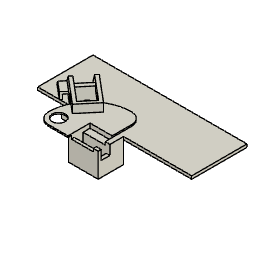
sorting_mechanism_platform (Autodesk Fusion 360 design; units mm, degrees)
Autodesk Fusion 360 part; units mm, degrees
note: some values were not read from the file. Set by a fixed rule: which sketch regions a step uses.
sketch "Sketch1" plane through (0, 0, 0) normal (0, 0, 1) x (1, 0, 0)
  line L0 (0, 0) -> (212, 0)
  line L1 (212, 0) -> (212, 78)
  line L2 (212, 78) -> (0, 78)
  line L3 (0, 78) -> (0, 0)
  dimension "d1" = 212
  dimension "d2" = 78
  constraint horizontal L0
  constraint vertical L1
  constraint horizontal L2
  constraint vertical L3
  constraint coincident L0.start L3.end
  measures "d1" distance of L0.start L0.end
  measures "d2" distance of L0.end L1.end
extrude "Extrude1" add sketch "Sketch1" along normal blind 4 makes body 1
sketch "Sketch2" plane through (0, 0, 4) normal (0, 0, 1) x (-1, 0, 0)
  line L0 (0, -78) -> (0, 0)
  line L1 (0, 0) -> (-212, 0)
  line L2 (-212, 0) -> (-212, -78)
  line L3 (-212, -78) -> (0, -78)
  line L4 (-31.7137, -41.9046) -> (-37.7137, -41.9046)
  line L5 (-37.7137, -41.9046) -> (-37.7137, -11.9046)
  line L6 (-37.7137, -11.9046) -> (-31.7137, -11.9046)
  line L7 (-31.7137, -11.9046) -> (-31.7137, -41.9046)
  dimension "d7" = 30
  dimension "d32" = 6
  constraint horizontal L4
  constraint vertical L5
  constraint horizontal L6
  constraint vertical L7
  measures "d7" distance of L4.start L6.end
  measures "d32" distance of L4.start L4.end
extrude "Extrude2" add sketch "Sketch2" along normal blind 12 contours L4 L5 L6 L7 bodies 1
sketch "Sketch4" plane through (0, 0, 16) normal (0, 0, 1) x (-1, 0, 0)
  line L0 (-31.7137, -11.9046) -> (-37.7137, -11.9046)
  line L1 (-37.7137, -11.9046) -> (-37.7137, -41.9046)
  line L2 (-37.7137, -41.9046) -> (-31.7137, -41.9046)
  line L3 (-31.7137, -41.9046) -> (-31.7137, -11.9046)
  line L4 (-31.7137, -41.9046) -> (-71.7137, -41.9046)
  line L5 (-71.7137, -41.9046) -> (-71.7137, -11.9046)
  line L6 (-71.7137, -11.9046) -> (-31.7137, -11.9046)
  line L7 (-31.7137, -11.9046) -> (-31.7137, -41.9046)
  dimension "d33" = 40
  constraint horizontal L4
  constraint vertical L5
  constraint horizontal L6
  constraint vertical L7
  constraint coincident L2.end L3.start
  constraint collinear L0 L6
  measures "d33" distance of L5 L7
extrude "Extrude3" add sketch "Sketch4" along normal blind 11 bodies 1
sketch "Sketch5" plane through (0, 0, 27) normal (0, 0, 1) x (-1, 0, 0)
  line L0 (-31.7137, -11.9046) -> (-71.7137, -11.9046)
  line L1 (-71.7137, -11.9046) -> (-71.7137, -41.9046)
  line L2 (-71.7137, -41.9046) -> (-31.7137, -41.9046)
  line L3 (-31.7137, -41.9046) -> (-31.7137, -11.9046)
  line L4 (-67.4138, -16.4046) -> (-37.7137, -16.4046)
  line L5 (-37.7137, -16.4046) -> (-37.7137, -37.4046)
  line L6 (-37.7137, -37.4046) -> (-67.4138, -37.4046)
  line L7 (-67.4138, -37.4046) -> (-67.4138, -16.4046)
  dimension "d14" = 21
  dimension "d15" = 4.5
  dimension "d34" = 6
  constraint horizontal L4
  constraint vertical L5
  constraint horizontal L6
  constraint vertical L7
  measures "d14" distance of L4.start L6.end
  measures "d15" distance of L2 L6
  measures "d34" distance of L3 L5
extrude "Extrude4" cut sketch "Sketch5" against normal blind 11 contours L4 L5 L6 L7 bodies 1
sketch "Sketch7" plane through (0, 0, 27) normal (0, 0, 1) x (-1, 0, 0)
  line L0 (-37.7137, -16.4046) -> (-37.7137, -37.4046)
  line L1 (-37.7137, -37.4046) -> (-67.4138, -37.4046)
  line L2 (-67.4138, -16.4046) -> (-37.7137, -16.4046)
  line L3 (-31.7137, -11.9046) -> (-71.7137, -11.9046)
  line L4 (-71.7137, -11.9046) -> (-71.7137, -41.9046)
  line L5 (-71.7137, -41.9046) -> (-31.7137, -41.9046)
  line L6 (-31.7137, -41.9046) -> (-31.7137, -11.9046)
  line L7 (-37.7137, -16.4046) -> (-31.7137, -16.4046)
  line L8 (-31.7137, -16.4046) -> (-31.7137, -37.4046)
  line L9 (-31.7137, -37.4046) -> (-37.7137, -37.4046)
  line L10 (-37.7137, -37.4046) -> (-37.7137, -16.4046)
  line L11 (-67.4138, -37.4046) -> (-67.4138, -16.4046)
  constraint horizontal L7
  constraint vertical L8
  constraint horizontal L9
  constraint vertical L10
  constraint coincident L6 L8.end
  constraint coincident L0.start L2.end
  constraint collinear L1 L9
extrude "Extrude5" cut sketch "Sketch7" against normal blind 4 contours L0 L6 L7 L8 L9 L10 bodies 1
sketch "Sketch8" plane through (0, 11.9046, 0) normal (0, -1, 0) x (1, 0, 0)
  line L0 (31.7137, 4) -> (37.7137, 4)
  line L1 (37.7137, 4) -> (37.7137, 16)
  line L2 (37.7137, 16) -> (71.7137, 16)
  line L3 (71.7137, 16) -> (71.7137, 27)
  line L4 (71.7137, 27) -> (31.7137, 27)
  line L5 (31.7137, 27) -> (31.7137, 4)
  line L6 (31.7137, 27) -> (24.7137, 27)
  line L7 (31.7137, 27) -> (31.7137, 4)
  line L8 (31.7137, 4) -> (4.7137, 4)
  line L9 (24.7137, 27) -> (4.7137, 4)
  dimension "d42" = 7
  dimension "d43" = 27
  constraint coincident L4.end L5.start
  constraint perpendicular L5 L6
  constraint coincident L0.start L5.end
  constraint perpendicular L7 L8
  measures "d42" distance of L4.end L6.end
  measures "d43" distance of L0.start L8.end
extrude "Extrude6" add sketch "Sketch8" against normal blind 4.5 contours L5 L6 L7 L8 L9 bodies 1
sketch "Sketch9" plane through (0, 41.9046, 0) normal (0, 1, 0) x (-1, 0, 0)
  line L0 (-37.7137, 4) -> (-31.7137, 4)
  line L1 (-31.7137, 4) -> (-31.7137, 27)
  line L2 (-31.7137, 27) -> (-71.7137, 27)
  line L3 (-71.7137, 27) -> (-71.7137, 16)
  line L4 (-71.7137, 16) -> (-37.7137, 16)
  line L5 (-37.7137, 16) -> (-37.7137, 4)
  line L6 (-31.7137, 27) -> (-24.7137, 27)
  line L7 (-31.7137, 27) -> (-31.7137, 4)
  line L8 (-31.7137, 4) -> (-4.7137, 4)
  line L9 (-24.7137, 27) -> (-4.7137, 4)
  dimension "d44" = 7
  dimension "d45" = 27
  constraint coincident L1.end L2.start
  constraint perpendicular L1 L6
  constraint coincident L0.end L1.start
  constraint perpendicular L1 L8
  measures "d44" distance of L1.end L6.end
  measures "d45" distance of L0.end L8.end
extrude "Extrude7" add sketch "Sketch9" against normal blind 4.5 contours L1 L6 L7 L8 L9 bodies 1
sketch "Sketch10" plane through (67.4138, 0, 0) normal (-1, 0, 0) x (0, -1, 0)
  line L0 (-16.4046, 27) -> (-37.4046, 27)
  line L1 (-37.4046, 27) -> (-37.4046, 16)
  line L2 (-16.4046, 16) -> (-16.4046, 27)
  line L3 (-29.9046, 25) -> (-23.9046, 25)
  line L4 (-23.9046, 25) -> (-23.9046, 22)
  line L5 (-23.9046, 22) -> (-29.9046, 22)
  line L6 (-29.9046, 22) -> (-29.9046, 27)
  line L7 (-37.4046, 16) -> (-16.4046, 16)
  dimension "d24" = 3
  dimension "d25" = 6
  dimension "d28" = 7.5
  dimension "d29" = 7.5
  dimension "d30" = 2
  constraint vertical L4
  constraint horizontal L5
  constraint vertical L6
  constraint coincident L0 L6.end
  constraint coincident L6 L3.start
  constraint perpendicular L3 L6
  measures "d24" distance of L3.end L4.end
  measures "d25" distance of L4.end L5.end
  measures "d28" distance of L1 L6
  measures "d29" distance of L2 L4
  measures "d30" distance of L0 L3
extrude "Extrude8" add sketch "Sketch10" along normal blind 4 contours L3 L4 L5 L6 bodies 1
sketch "Sketch11" plane through (0, 0, 4) normal (0, 0, 1) x (-1, 0, 0)
  line L0 (-31.7137, -37.4046) -> (-4.7137, -37.4046)
  line L1 (-4.7137, -37.4046) -> (-4.7137, -41.9046)
  line L2 (-4.7137, -41.9046) -> (-37.7137, -41.9046)
  line L3 (-37.7137, -41.9046) -> (-37.7137, -11.9046)
  line L4 (-37.7137, -11.9046) -> (-4.7137, -11.9046)
  line L5 (-4.7137, -11.9046) -> (-4.7137, -16.4046)
  line L6 (-4.7137, -16.4046) -> (-31.7137, -16.4046)
  line L7 (-31.7137, -16.4046) -> (-31.7137, -37.4046)
  line L8 (0, -78) -> (0, 0)
  line L9 (0, 0) -> (-212, 0)
  line L10 (-212, 0) -> (-212, -78)
  line L11 (-212, -78) -> (0, -78)
  circle A0 centre (-98, -18.5) radius 10
  dimension "d46" = 20
  dimension "d47" = 59.5
  dimension "d50" = 114
  measures "d46" diameter of A0
  measures "d47" distance of L11 A0.centre
  measures "d50" distance of L10 A0.centre
extrude "Extrude9" add sketch "Sketch11" along normal blind 2 contours A0 bodies 1
sketch "Sketch12" plane through (0, 0, 0) normal (0, 0, -1) x (1, 0, 0)
  line L0 (0, 0) -> (0, -78)
  line L1 (0, -78) -> (212, -78)
  line L2 (212, -78) -> (212, 0)
  line L3 (212, 0) -> (0, 0)
  line L4 (77.5, 0) -> (118.5, 0)
  line L5 (118.5, 0) -> (118.5, -4)
  line L6 (118.5, -4) -> (77.5, -4)
  line L7 (77.5, -4) -> (77.5, 0)
  circle A0 centre (98, -18.5) radius 10
  dimension "d60" = 4
  dimension "d66" = 20.5
  dimension "d67" = 41
  constraint horizontal L4
  constraint vertical L5
  constraint horizontal L6
  constraint vertical L7
  constraint coincident L3 L4.start
  measures "d60" distance of L4.end L5.end
  measures "d66" distance of L5 A0.centre
  measures "d67" distance of L5.end L6.end
extrude "Extrude10" add sketch "Sketch12" along normal blind 29 contours L3 L4 L5 L6 L7 bodies 1
sketch "Sketch18" plane through (0, 0, 0) normal (0, -1, 0) x (1, 0, 0)
  line L0 (0, 0) -> (77.5, 0)
  line L1 (77.5, 0) -> (77.5, -29)
  line L2 (77.5, -29) -> (118.5, -29)
  line L3 (118.5, -29) -> (118.5, 0)
  line L4 (118.5, 0) -> (212, 0)
  line L5 (212, 0) -> (212, 4)
  line L6 (212, 4) -> (0, 4)
  line L7 (0, 4) -> (0, 0)
  line L8 (77.5, -29) -> (118.5, -29)
  line L9 (118.5, -29) -> (118.5, -25)
  line L10 (118.5, -25) -> (77.5, -25)
  line L11 (77.5, -25) -> (77.5, -29)
  dimension "d61" = 4
  constraint horizontal L8
  constraint vertical L9
  constraint horizontal L10
  constraint vertical L11
  constraint coincident L3 L9.end
  constraint coincident L1.end L2.start
  measures "d61" distance of L2.end L9.end
extrude "Extrude14" add sketch "Sketch18" along normal blind 30.5 contours L1 L2 L3 L8 L9 L10 L11 bodies 1
sketch "Sketch19" plane through (118.5, 0, 0) normal (1, 0, 0) x (0, 1, 0)
  line L0 (4, 0) -> (0, 0)
  line L1 (0, 0) -> (0, -25)
  line L2 (0, -25) -> (-30.5, -25)
  line L3 (-30.5, -25) -> (-30.5, -29)
  line L4 (-30.5, -29) -> (4, -29)
  line L5 (4, -29) -> (4, 0)
  line L6 (-30.5, -25) -> (0, -25)
  line L7 (0, -25) -> (0, 4)
  line L8 (0, 4) -> (-30.5, 4)
  line L9 (-30.5, 4) -> (-30.5, -25)
  line L10 (-30.5, -25) -> (0, -25)
  line L11 (0, -25) -> (0, 4)
  constraint coincident L2.end L3.start
  constraint coincident L1.end L2.start
  constraint perpendicular L0 L7
  constraint horizontal L8
  constraint vertical L9
  constraint horizontal L10
  constraint vertical L11
extrude "Extrude15" add sketch "Sketch19" against normal blind 41 contours L1 L2 L6 L7 L8 L9 L10 L11 bodies 1
sketch "Sketch21" plane through (0, 0, 4) normal (0, 0, 1) x (-1, 0, 0)
  circle A0 centre (-98, -18.5) radius 10
  line L0 (-31.7137, -37.4046) -> (-4.7137, -37.4046)
  line L1 (-4.7137, -37.4046) -> (-4.7137, -41.9046)
  line L2 (-4.7137, -41.9046) -> (-37.7137, -41.9046)
  line L3 (-37.7137, -41.9046) -> (-37.7137, -11.9046)
  line L4 (-37.7137, -11.9046) -> (-4.7137, -11.9046)
  line L5 (-4.7137, -11.9046) -> (-4.7137, -16.4046)
  line L6 (-4.7137, -16.4046) -> (-31.7137, -16.4046)
  line L7 (-31.7137, -16.4046) -> (-31.7137, -37.4046)
  line L8 (0, -78) -> (0, 0)
  line L9 (0, 0) -> (-77.5, 0)
  line L10 (-212, 0) -> (-212, -78)
  line L11 (-212, -78) -> (0, -78)
  circle A1 centre (-98, 24) radius 56.5
  line L12 (-98, 24) -> (-113, 24)
  line L13 (-113, 24) -> (-113, -32.5)
  line L14 (-113, -32.5) -> (-98, -32.5)
  line L15 (-98, -32.5) -> (-98, 24)
  line L16 (-98, 24) -> (-41.5, 24)
  line L17 (-41.5, 24) -> (-41.5, 39)
  line L18 (-41.5, 39) -> (-98, 39)
  line L19 (-98, 39) -> (-98, 24)
  line L20 (-113, 24) -> (-98, 24)
  line L21 (-98, 24) -> (-98, 39)
  line L22 (-98, 39) -> (-113, 39)
  line L23 (-113, 39) -> (-113, 24)
  line L24 (-77.5, 0) -> (-77.5, 30.5)
  line L25 (-77.5, 30.5) -> (-118.5, 30.5)
  line L26 (-118.5, 30.5) -> (-118.5, 0)
  line L27 (-118.5, 0) -> (-212, 0)
  dimension "d72" = 114
  dimension "d73" = 114
  dimension "d74" = 113
  dimension "d75" = 42.5
  dimension "d76" = 56.5
  dimension "d77" = 56.5
  dimension "d78" = 15
  dimension "d79" = 15
  constraint horizontal L12
  constraint vertical L13
  constraint horizontal L14
  constraint vertical L15
  constraint coincident A1.centre L12.start
  constraint horizontal L16
  constraint vertical L17
  constraint horizontal L18
  constraint vertical L19
  constraint horizontal L20
  constraint vertical L21
  constraint horizontal L22
  constraint vertical L23
  measures "d72" distance of A0.centre L10
  measures "d73" distance of L10 A1.centre
  measures "d74" diameter of A1
  measures "d75" distance of A0.centre A1.centre
  measures "d76" distance of L12.end L13.end
  measures "d77" distance of L17.end L18.end
  measures "d78" distance of L13.end L14.end
  measures "d79" distance of L16.end L17.end
extrude "Extrude17" add sketch "Sketch21" along normal blind 2 contours A0 L9 A1 L15 L16 L24 | A0 A1 L12 L13 L15 L20 | L16 L19 L21 L24 L25 | L12 L19 L20 L21 L23 L25 | A1 L13 L14 | A1 L16 L18 L19 L21 L24 L25 | L9 A1 L16 L24 | L19 L21 L22 L23 L25 | A1 L17 L18 bodies 1
fillet "Fillet1" radius 15 2 edges at (41.5, -39, 5) (113, 32.5, 5) on bodies 1
sketch "Sketch22" plane through (0, 0, 6) normal (0, 0, 1) x (-1, 0, 0)
  arc A0 (-113, -17.5) -> (-98, -32.5) centre (-98, -17.5) ccw
  arc A1 (-98, -32.5) -> (-41.5, 24) centre (-98, 24) ccw
  arc A2 (-41.5, 24) -> (-56.5, 39) centre (-56.5, 24) ccw
  line L0 (-56.5, 39) -> (-113, 39)
  line L1 (-113, 39) -> (-113, -17.5)
  line L2 (-113, 0) -> (-83, 0)
  line L3 (-83, 0) -> (-83, 39)
  line L4 (-83, 39) -> (-113, 39)
  line L5 (-113, 39) -> (-113, 0)
  line L6 (-77.5, -4) -> (-118.5, -4)
  line L7 (-118.5, -4) -> (-118.5, 30.5)
  line L8 (-118.5, 30.5) -> (-77.5, 30.5)
  line L9 (-77.5, 30.5) -> (-77.5, -4)
  line L10 (-113, -17.5) -> (-113, 30.5)
  line L11 (-118.5, 0) -> (-212, 0)
  line L12 (-212, 0) -> (-212, -78)
  line L13 (-212, -78) -> (0, -78)
  line L14 (0, -78) -> (0, 0)
  line L15 (0, 0) -> (-46.8507, 0)
  arc A3 (-98, -32.5) -> (-46.8507, 0) centre (-98, 24) ccw
  arc A4 (-113, -17.5) -> (-98, -32.5) centre (-98, -17.5) ccw
  line L16 (-31.7137, -37.4046) -> (-4.7137, -37.4046)
  line L17 (-4.7137, -37.4046) -> (-4.7137, -41.9046)
  line L18 (-4.7137, -41.9046) -> (-37.7137, -41.9046)
  line L19 (-37.7137, -41.9046) -> (-37.7137, -11.9046)
  line L20 (-37.7137, -11.9046) -> (-4.7137, -11.9046)
  line L21 (-4.7137, -11.9046) -> (-4.7137, -16.4046)
  line L22 (-4.7137, -16.4046) -> (-31.7137, -16.4046)
  line L23 (-31.7137, -16.4046) -> (-31.7137, -37.4046)
  line L24 (0, 0) -> (-46.8507, 0)
  line L25 (-118.5, 0) -> (-212, 0)
  line L26 (-113, 30.5) -> (-118.5, 30.5)
  line L27 (-118.5, 30.5) -> (-118.5, 0)
  line L28 (-83, 0) -> (-118.5, 0)
  line L29 (-118.5, 0) -> (-118.5, 9)
  line L30 (-118.5, 9) -> (-83, 9)
  line L31 (-83, 9) -> (-83, 0)
  dimension "d84" = 32.5
  dimension "d95" = 5.5
  dimension "d112" = 9
  constraint horizontal L2
  constraint horizontal L4
  constraint vertical L5
  constraint coincident L0 L3.end
  constraint coincident L1 L2.start
  constraint horizontal L28
  constraint vertical L29
  constraint horizontal L30
  constraint vertical L31
  constraint coincident L7 L29.end
  measures "d84" distance of A0.end L2
  measures "d95" distance of L3 L9
  measures "d112" distance of L2 L30
extrude "Extrude18" cut sketch "Sketch22" against normal blind 2 contours L1 L3 L5 L8 L10 L30 | L0 L1 L3 L4 L5 L8 bodies 1
sketch "Sketch23" plane through (0, 0, 6) normal (0, 0, 1) x (-1, 0, 0)
  line L0 (-83, 39) -> (-83, 9)
  line L1 (-113, 9) -> (-113, -17.5)
  arc A0 (-113, -17.5) -> (-98, -32.5) centre (-98, -17.5) ccw
  arc A1 (-98, -32.5) -> (-41.5, 24) centre (-98, 24) ccw
  arc A2 (-41.5, 24) -> (-56.5, 39) centre (-56.5, 24) ccw
  line L2 (-56.5, 39) -> (-83, 39)
  circle A3 centre (-55.5, 24) radius 9
  line L3 (-83, 9) -> (-113, 9)
  dimension "d89" = 18
  dimension "d90" = 15
  dimension "d91" = 14
  measures "d89" diameter of A3
  measures "d90" distance of L2 A3.centre
  measures "d91" distance of A1.end A3.centre
extrude "Extrude19" cut sketch "Sketch23" against normal blind 2 contours A3 bodies 1
sketch "Sketch24" plane through (0, 0, 4) normal (0, 0, 1) x (-1, 0, 0)
  line L0 (-113, -17.5) -> (-113, 9)
  line L1 (-83, 9) -> (-83, 30.5)
  line L2 (-83, 30.5) -> (-118.5, 30.5)
  line L3 (-118.5, 30.5) -> (-118.5, 0)
  line L4 (-118.5, 0) -> (-212, 0)
  line L5 (-212, 0) -> (-212, -78)
  line L6 (-212, -78) -> (0, -78)
  line L7 (0, -78) -> (0, 0)
  line L8 (0, 0) -> (-46.8507, 0)
  arc A0 (-98, -32.5) -> (-46.8507, 0) centre (-98, 24) ccw
  arc A1 (-113, -17.5) -> (-98, -32.5) centre (-98, -17.5) ccw
  line L9 (-31.7137, -37.4046) -> (-4.7137, -37.4046)
  line L10 (-4.7137, -37.4046) -> (-4.7137, -41.9046)
  line L11 (-4.7137, -41.9046) -> (-37.7137, -41.9046)
  line L12 (-37.7137, -41.9046) -> (-37.7137, -11.9046)
  line L13 (-37.7137, -11.9046) -> (-4.7137, -11.9046)
  line L14 (-4.7137, -11.9046) -> (-4.7137, -16.4046)
  line L15 (-4.7137, -16.4046) -> (-31.7137, -16.4046)
  line L16 (-31.7137, -16.4046) -> (-31.7137, -37.4046)
  line L17 (-83, 30.5) -> (-114.5, 30.5)
  line L18 (-114.5, 30.5) -> (-114.5, 18.5)
  line L19 (-114.5, 18.5) -> (-83, 18.5)
  line L20 (-83, 18.5) -> (-83, 30.5)
  line L21 (-113, 9) -> (-83, 9)
  dimension "d96" = 4
  dimension "d98" = 12
  constraint horizontal L17
  constraint vertical L18
  constraint horizontal L19
  constraint vertical L20
  constraint coincident L2 L1.end
  constraint collinear L1 L20
  measures "d96" distance of L3 L18
  measures "d98" distance of L17.end L18.end
extrude "Extrude20" cut sketch "Sketch24" against normal blind 29 contours L1 L2 L17 L18 L19 L20 bodies 1
sketch "Sketch25" plane through (0, -30.5, 0) normal (0, -1, 0) x (1, 0, 0)
  line L0 (83, -25) -> (83, 4)
  line L1 (83, 4) -> (77.5, 4)
  line L2 (77.5, 4) -> (77.5, -29)
  line L3 (77.5, -29) -> (118.5, -29)
  line L4 (118.5, -29) -> (118.5, 4)
  line L5 (118.5, 4) -> (114.5, 4)
  line L6 (114.5, 4) -> (114.5, -25)
  line L7 (114.5, -25) -> (83, -25)
  line L8 (77.5, -29) -> (118.5, -29)
  line L9 (118.5, -29) -> (118.5, 4)
  line L10 (118.5, 4) -> (77.5, 4)
  line L11 (77.5, 4) -> (77.5, -29)
  constraint horizontal L8
  constraint vertical L9
  constraint horizontal L10
  constraint vertical L11
  constraint coincident L4.end L5.start
  constraint coincident L2.end L3.start
extrude "Extrude21" add sketch "Sketch25" along normal blind 4 bodies 1
sketch "Sketch26" plane through (0, 0, 4) normal (0, 0, 1) x (-1, 0, 0)
  line L0 (-31.7137, -37.4046) -> (-4.7137, -37.4046)
  line L1 (-4.7137, -37.4046) -> (-4.7137, -41.9046)
  line L2 (-4.7137, -41.9046) -> (-37.7137, -41.9046)
  line L3 (-37.7137, -41.9046) -> (-37.7137, -11.9046)
  line L4 (-37.7137, -11.9046) -> (-4.7137, -11.9046)
  line L5 (-4.7137, -11.9046) -> (-4.7137, -16.4046)
  line L6 (-4.7137, -16.4046) -> (-31.7137, -16.4046)
  line L7 (-31.7137, -16.4046) -> (-31.7137, -37.4046)
  line L8 (-83, 18.5) -> (-114.5, 18.5)
  line L9 (-114.5, 18.5) -> (-114.5, 30.5)
  line L10 (-114.5, 30.5) -> (-83, 30.5)
  line L11 (-83, 30.5) -> (-83, 34.5)
  line L12 (-83, 34.5) -> (-118.5, 34.5)
  line L13 (-118.5, 34.5) -> (-118.5, 0)
  line L14 (-118.5, 0) -> (-212, 0)
  line L15 (-212, 0) -> (-212, -78)
  line L16 (-212, -78) -> (0, -78)
  line L17 (0, -78) -> (0, 0)
  line L18 (0, 0) -> (-46.8507, 0)
  arc A0 (-98, -32.5) -> (-46.8507, 0) centre (-98, 24) ccw
  arc A1 (-113, -17.5) -> (-98, -32.5) centre (-98, -17.5) ccw
  line L19 (-113, -17.5) -> (-113, 9)
  line L20 (-83, 9) -> (-83, 18.5)
  line L21 (-114.5, 18.5) -> (-118.5, 18.5)
  line L22 (-118.5, 18.5) -> (-118.5, 30.5)
  line L23 (-118.5, 30.5) -> (-114.5, 30.5)
  line L24 (-114.5, 30.5) -> (-114.5, 18.5)
  line L25 (-113, 9) -> (-83, 9)
  constraint horizontal L21
  constraint vertical L22
  constraint horizontal L23
  constraint vertical L24
  constraint coincident L13 L22.end
  constraint coincident L8.end L9.start
  constraint collinear L10 L23
extrude "Extrude22" cut sketch "Sketch26" against normal blind 13 contours L9 L13 L21 L22 L23 L24 bodies 1
extrude "Extrude25" add 1 faces at (118.5, -16.3333, -22.3333) along direction (1, 0, 0) blind 1 on bodies 1 bodies 1
sketch "Sketch29" plane through (0, 0, 4) normal (0, 0, 1) x (-1, 0, 0)
  line L0 (-83, 18.5) -> (-119.5, 18.5)
  line L1 (-119.5, 18.5) -> (-119.5, 0)
  line L2 (-119.5, 0) -> (-212, 0)
  line L3 (-212, 0) -> (-212, -78)
  line L4 (-212, -78) -> (0, -78)
  line L5 (0, -78) -> (0, 0)
  line L6 (0, 0) -> (-46.8507, 0)
  arc A0 (-98, -32.5) -> (-46.8507, 0) centre (-98, 24) ccw
  arc A1 (-113, -17.5) -> (-98, -32.5) centre (-98, -17.5) ccw
  line L7 (-113, -17.5) -> (-113, 9)
  line L8 (-113, 9) -> (-83, 9)
  line L9 (-83, 9) -> (-83, 18.5)
  line L10 (-31.7137, -37.4046) -> (-4.7137, -37.4046)
  line L11 (-4.7137, -37.4046) -> (-4.7137, -41.9046)
  line L12 (-4.7137, -41.9046) -> (-37.7137, -41.9046)
  line L13 (-37.7137, -41.9046) -> (-37.7137, -11.9046)
  line L14 (-37.7137, -11.9046) -> (-4.7137, -11.9046)
  line L15 (-4.7137, -11.9046) -> (-4.7137, -16.4046)
  line L16 (-4.7137, -16.4046) -> (-31.7137, -16.4046)
  line L17 (-31.7137, -16.4046) -> (-31.7137, -37.4046)
  line L18 (-83, 9) -> (-113, 9)
  line L19 (-113, 9) -> (-113, 34.5)
  line L20 (-113, 34.5) -> (-83, 34.5)
  line L21 (-83, 34.5) -> (-83, 9)
  line L22 (-83, 34.5) -> (-119.5, 34.5)
  constraint horizontal L18
  constraint vertical L19
  constraint horizontal L20
  constraint vertical L21
  constraint coincident L8.end L9.start
  constraint collinear L20 L22
  constraint collinear L7 L19
extrude "Extrude26" cut sketch "Sketch29" against normal blind 4 contours L0 L8 L9 L18 L19 L21 | L0 L19 L20 L21 L22 bodies 1
extrude "Extrude27" cut 1 faces at (77.5, -23, -8.3333) along direction (1, 0, 0) blind 1.5 on bodies 1 bodies 1
sketch "Sketch30" plane through (79, 0, 0) normal (-1, 0, 0) x (0, -1, 0)
  line L0 (0, 0) -> (-4, 0)
  line L1 (-4, 0) -> (-4, -29)
  line L2 (-4, -29) -> (34.5, -29)
  line L3 (34.5, -29) -> (34.5, 4)
  line L4 (34.5, 4) -> (0, 4)
  line L5 (0, 4) -> (0, 0)
  line L6 (30.5, 0) -> (30.5, -25)
  line L7 (30.5, -25) -> (18.5, -25)
  line L8 (18.5, -25) -> (18.5, 0)
  line L9 (18.5, 0) -> (9, 0)
  line L10 (9, 0) -> (9, 6)
  line L11 (9, 6) -> (39, 6)
  line L12 (39, 6) -> (39, 4)
  line L13 (39, 4) -> (34.5, 4)
  line L14 (34.5, 4) -> (34.5, 0)
  line L15 (34.5, 0) -> (30.5, 0)
  line L16 (18.5, -25) -> (30.5, -25)
  line L17 (30.5, -25) -> (30.5, -15)
  line L18 (30.5, -15) -> (18.5, -15)
  line L19 (18.5, -15) -> (18.5, -25)
  dimension "d117" = 10
  constraint horizontal L16
  constraint vertical L17
  constraint horizontal L18
  constraint vertical L19
  constraint coincident L6 L17.end
  constraint coincident L7.end L8.start
  measures "d117" distance of L16 L18
extrude "Extrude28" cut sketch "Sketch30" against normal blind 4 contours L6 L7 L8 L16 L17 L18 L19 bodies 1
sketch "Sketch31" plane through (0, 0, -29) normal (0, 0, -1) x (1, 0, 0)
  line L0 (79, 34.5) -> (79, -4)
  line L1 (79, -4) -> (119.5, -4)
  line L2 (119.5, -4) -> (119.5, 34.5)
  line L3 (119.5, 34.5) -> (79, 34.5)
  line L4 (79, 30.5) -> (114.5, 30.5)
  line L5 (114.5, 30.5) -> (114.5, 18.5)
  line L6 (114.5, 18.5) -> (79, 18.5)
  line L7 (79, 18.5) -> (79, 30.5)
  line L8 (83, -4) -> (114.5, -4)
  line L9 (114.5, -4) -> (114.5, 14.5)
  line L10 (114.5, 14.5) -> (83, 14.5)
  line L11 (83, 14.5) -> (83, -4)
  dimension "d120" = 4
  dimension "d121" = 5
  dimension "d122" = 4
  constraint horizontal L8
  constraint vertical L9
  constraint horizontal L10
  constraint vertical L11
  constraint coincident L1 L8.start
  measures "d120" distance of L0 L11
  measures "d121" distance of L2 L9
  measures "d122" distance of L6 L10
extrude "Extrude29" cut sketch "Sketch31" against normal blind 25 contours L1 L8 L9 L10 L11 bodies 1
copy_body "CopyPasteBodies1" bodies 1 makes body 2
move_body "Move1" bodies 2 to x (1, 0, 0) y (0, 1, 0) z (0, 0, 1) at (0, 0, 0)
sketch "Sketch32" plane through (0, 0, 0) normal (0, -1, 0) x (1, 0, 0)
  line L0 (79, 4) -> (46.8507, 4)
  line L1 (46.8507, 4) -> (0, 4)
  line L2 (0, 4) -> (0, 0)
  line L3 (0, 0) -> (79, 0)
  line L4 (79, 0) -> (79, 4)
  line L5 (0, 4) -> (212, 4)
  line L6 (212, 4) -> (212, -29)
  line L7 (212, -29) -> (0, -29)
  line L8 (0, -29) -> (0, 4)
  line L9 (79, -29) -> (119.5, -29)
  line L10 (212, 0) -> (212, 4)
  line L11 (41.5, 4) -> (113, 4)
  line L12 (113, 4) -> (113, 6)
  line L13 (113, 6) -> (41.5, 6)
  line L14 (41.5, 6) -> (41.5, 4)
  line L15 (56.5, 6) -> (83, 6)
  line L16 (41.5, 4) -> (41.5, 6)
  line L17 (113, 6) -> (113, 4)
  constraint horizontal L5
  constraint vertical L6
  constraint horizontal L7
  constraint vertical L8
  constraint coincident L1.end L2.start
  constraint collinear L7 L9
  constraint collinear L6 L10
  constraint horizontal L11
  constraint vertical L12
  constraint horizontal L13
  constraint vertical L14
  constraint coincident L5 L11.start
  constraint collinear L13 L15
  constraint collinear L14 L16
  constraint collinear L12 L17
extrude "Extrude30" cut sketch "Sketch32" along normal blind 39 and the other way blind 78 bodies 2
move_body "Move2" bodies 2 to x (0.766044, -0.642788, 0) y (0.642788, 0.766044, 0) z (0, 0, 1) at (7.2782, 17.1601, 0)
extrude "Extrude31" cut 1 faces at (22.3804, 11.9046, 11.6667) along direction (0, 1, 0) blind 30 on bodies 1 bodies 1
sketch "Sketch33" plane through (0, 0, -29) normal (0, 0, -1) x (1, 0, 0)
  line L0 (83, -4) -> (83, 14.5)
  line L1 (83, 14.5) -> (114.5, 14.5)
  line L2 (114.5, 14.5) -> (114.5, -4)
  line L3 (114.5, -4) -> (119.5, -4)
  line L4 (119.5, -4) -> (119.5, 34.5)
  line L5 (119.5, 34.5) -> (79, 34.5)
  line L6 (79, 34.5) -> (79, -4)
  line L7 (79, -4) -> (83, -4)
  line L8 (119.5, -4) -> (79, -4)
  line L9 (79, -4) -> (79, 0)
  line L10 (79, 0) -> (119.5, 0)
  line L11 (119.5, 0) -> (119.5, -4)
  dimension "d131" = 4
  constraint horizontal L8
  constraint vertical L9
  constraint horizontal L10
  constraint vertical L11
  constraint coincident L6 L9.end
  constraint coincident L3.end L4.start
  measures "d131" distance of L8 L10
extrude "Extrude32" cut sketch "Sketch33" against normal blind 29 contours L0 L6 L7 L8 L9 L10 | L0 L2 L8 L10 | L2 L3 L4 L8 L10 L11 bodies 1
sketch "Sketch34" plane through (0, 0, 4) normal (0, 0, 1) x (-1, 0, 0)
  line L0 (-113, 9) -> (-113, 18.5)
  line L1 (-113, 18.5) -> (-119.5, 18.5)
  line L2 (-119.5, 18.5) -> (-119.5, 0)
  line L3 (-119.5, 0) -> (-212, 0)
  line L4 (-212, 0) -> (-212, -78)
  line L5 (-212, -78) -> (0, -78)
  line L6 (0, -78) -> (0, 0)
  line L7 (0, 0) -> (-46.8507, 0)
  arc A0 (-98, -32.5) -> (-46.8507, 0) centre (-98, 24) ccw
  arc A1 (-113, -17.5) -> (-98, -32.5) centre (-98, -17.5) ccw
  line L8 (-113, -17.5) -> (-113, 9)
  line L9 (-14.6845, -18.6534) -> (-34.1616, -2.3102)
  line L10 (-34.1616, -2.3102) -> (-32.2332, -0.012)
  line L11 (-32.2332, -0.012) -> (-12.7561, -16.3553)
  line L12 (-12.7561, -16.3553) -> (-14.6845, -18.6534)
  line L13 (-33.8621, -10.3939) -> (-18.5412, -23.2497)
  line L14 (-33.8621, -10.3939) -> (-36.7546, -13.8411)
  line L15 (-18.5412, -23.2497) -> (-21.4337, -26.6969)
  dimension "d134" = 3
  dimension "d138" = 6
  constraint perpendicular L9 L10
  constraint perpendicular L10 L11
  constraint parallel L9 L13
  constraint parallel L12 L14
  constraint collinear L12 L15
  measures "d134" distance of L9.end L10.end
  measures "d138" distance of L9 L13
extrude "Extrude33" add sketch "Sketch34" along normal blind 9 contours L9 L10 L11 L12 bodies 1
sketch "Sketch35" plane through (15.2523, 18.177, 0) normal (0.642788, 0.766044, 0) x (-0.766044, 0.642788, 0)
  line L0 (-24.6844, 4) -> (0.7412, 4)
  line L1 (0.7412, 4) -> (0.7412, 13)
  line L2 (0.7412, 13) -> (-24.6844, 13)
  line L3 (-24.6844, 13) -> (-24.6844, 4)
  line L4 (-24.6844, 13) -> (0.7412, 13)
  line L5 (0.7412, 13) -> (0.7412, 10)
  line L6 (0.7412, 10) -> (-24.6844, 10)
  line L7 (-24.6844, 10) -> (-24.6844, 13)
  dimension "d139" = 3
  constraint horizontal L4
  constraint vertical L5
  constraint horizontal L6
  constraint vertical L7
  constraint coincident L1 L5.end
  constraint coincident L2.end L3.start
  measures "d139" distance of L4 L6
extrude "Extrude34" add sketch "Sketch35" along normal blind 6 contours L1 L2 L3 L4 L5 L6 L7 bodies 1 2
sketch "Sketch36" plane through (13.3239, 15.8788, 0) normal (-0.642788, -0.766044, 0) x (0.766044, -0.642788, 0)
  line L0 (-0.7412, 4) -> (24.6844, 4)
  line L1 (24.6844, 4) -> (24.6844, 13)
  line L2 (24.6844, 13) -> (-0.7412, 13)
  line L3 (-0.7412, 13) -> (-0.7412, 4)
  line L4 (24.6844, 10) -> (4.4762, 10)
  line L5 (4.4762, 10) -> (-0.7412, 4)
  line L6 (-0.7412, 4) -> (32.2588, 4)
  line L7 (32.2588, 4) -> (32.2588, 16)
  line L8 (32.2588, 16) -> (66.2588, 16)
  line L9 (66.2588, 16) -> (66.2588, 27)
  line L10 (66.2588, 27) -> (19.2588, 27)
  line L11 (19.2588, 27) -> (7.0849, 13)
  line L12 (7.0849, 13) -> (24.6844, 13)
  line L13 (24.6844, 13) -> (24.6844, 10)
  line L14 (-0.7412, 4) -> (7.0849, 13)
  line L15 (-0.7412, 13) -> (7.0849, 13)
  line L16 (-0.7412, 13) -> (-0.7412, 4)
  constraint coincident L0.start L3.end
  constraint coincident L11.end L12.start
  constraint coincident L2.end L3.start
extrude "Extrude35" cut sketch "Sketch36" against normal blind 9 contours L2 L3 L5 L14 L15 L16 bodies 1
sketch "Sketch37" plane through (0, 0, 4) normal (0, 0, -1) x (1, 0, 0)
  line L0 (79, 34.5) -> (83, 34.5)
  line L1 (83, 34.5) -> (83, 39)
  line L2 (83, 39) -> (56.5, 39)
  arc A0 (56.5, 39) -> (41.5, 24) centre (56.5, 24) ccw
  arc A1 (41.5, 24) -> (46.8507, 0) centre (98, 24) ccw
  line L3 (46.8507, 0) -> (79, 0)
  line L4 (79, 0) -> (79, 34.5)
  circle A2 centre (55.5, 24) radius 9
  line L5 (47, 0) -> (69, 0)
  line L6 (69, 0) -> (69, 3)
  line L7 (69, 3) -> (47, 3)
  line L8 (47, 3) -> (47, 0)
  line L9 (47, 12) -> (69, 12)
  line L10 (69, 12) -> (69, 9)
  line L11 (69, 9) -> (47, 9)
  line L12 (47, 9) -> (47, 12)
  dimension "d144" = 3
  dimension "d145" = 3
  dimension "d146" = 6
  dimension "d151" = 10
  dimension "d152" = 22
  constraint horizontal L5
  constraint vertical L6
  constraint horizontal L7
  constraint vertical L8
  constraint coincident L3 L5.start
  constraint horizontal L9
  constraint vertical L10
  constraint horizontal L11
  constraint vertical L12
  constraint collinear L6 L10
  constraint collinear L8 L12
  measures "d144" distance of L9.end L10.end
  measures "d145" distance of L5.end L6.end
  measures "d146" distance of L7 L11
  measures "d151" distance of L4 L6
  measures "d152" distance of L6 L8
extrude "Extrude36" add sketch "Sketch37" along normal blind 9 contours L3 L5 L6 L7 L8 | L9 L10 L11 L12 bodies 1
sketch "Sketch38" plane through (0, 0, -5) normal (0, 0, -1) x (1, 0, 0)
  line L0 (47, 9) -> (69, 9)
  line L1 (69, 9) -> (69, 12)
  line L2 (69, 12) -> (47, 12)
  line L3 (47, 12) -> (47, 9)
  line L4 (47, 12) -> (69, 12)
  line L5 (69, 12) -> (69, 0)
  line L6 (69, 0) -> (47, 0)
  line L7 (47, 0) -> (47, 12)
  constraint horizontal L4
  constraint vertical L5
  constraint horizontal L6
  constraint vertical L7
  constraint coincident L2.end L3.start
  constraint collinear L1 L5
extrude "Extrude37" add sketch "Sketch38" against normal blind 3 bodies 1
sketch "Sketch39" plane through (0, 0, 4) normal (0, 0, 1) x (-1, 0, 0)
  line L0 (-14.6845, -18.6534) -> (-34.1616, -2.3102)
  line L1 (-34.1616, -2.3102) -> (-32.2332, -0.012)
  line L2 (-32.2332, -0.012) -> (-12.7561, -16.3553)
  line L3 (-12.7561, -16.3553) -> (-14.6845, -18.6534)
  line L4 (-18.5412, -23.2497) -> (-21.4337, -26.6969)
  line L5 (-21.4337, -26.6969) -> (-42.1169, -9.3416)
  line L6 (-42.1169, -9.3416) -> (-55.6155, -25.4286)
  line L7 (-55.6155, -25.4286) -> (-34.9323, -42.7838)
  line L8 (-34.9323, -42.7838) -> (-37.8248, -46.231)
  line L9 (-37.8248, -46.231) -> (-63.1043, -25.019)
  line L10 (-63.1043, -25.019) -> (-43.8207, -2.0377)
  line L11 (-43.8207, -2.0377) -> (-18.5412, -23.2497)
  line L12 (-113, 9) -> (-113, 18.5)
  line L13 (-113, 18.5) -> (-119.5, 18.5)
  line L14 (-119.5, 18.5) -> (-119.5, 0)
  line L15 (-119.5, 0) -> (-212, 0)
  line L16 (-212, 0) -> (-212, -78)
  line L17 (-212, -78) -> (0, -78)
  line L18 (0, -78) -> (0, 0)
  line L19 (0, 0) -> (-46.8507, 0)
  arc A0 (-98, -32.5) -> (-46.8507, 0) centre (-98, 24) ccw
  arc A1 (-113, -17.5) -> (-98, -32.5) centre (-98, -17.5) ccw
  line L20 (-113, -17.5) -> (-113, 9)
  line L21 (-212, -78) -> (0, -78)
  line L22 (0, -78) -> (0, -75)
  line L23 (0, -75) -> (-212, -75)
  line L24 (-212, -75) -> (-212, -78)
  line L25 (0, 0) -> (-3, 0)
  line L26 (-3, 0) -> (-3, -75)
  line L27 (-3, -75) -> (0, -75)
  line L28 (0, -75) -> (0, 0)
  dimension "d153" = 3
  dimension "d154" = 3
  constraint horizontal L21
  constraint vertical L22
  constraint horizontal L23
  constraint vertical L24
  constraint coincident L18 L22.end
  constraint coincident L16.end L17.start
  constraint horizontal L25
  constraint vertical L26
  constraint horizontal L27
  constraint vertical L28
  constraint coincident L23 L26.end
  constraint coincident L18.end L19.start
  measures "d153" distance of L21 L23
  measures "d154" distance of L26 L28
extrude "Extrude38" cut sketch "Sketch39" against normal blind 4 contours L18 L19 L23 L25 L26 L27 L28 | L16 L17 L18 L21 L22 L23 L24 L27 bodies 1
sketch "Sketch40" plane through (79, 0, 0) normal (-1, 0, 0) x (0, -1, 0)
  line L0 (0, 0) -> (0, -29)
  line L1 (0, -29) -> (34.5, -29)
  line L2 (34.5, -29) -> (34.5, 4)
  line L3 (34.5, 4) -> (0, 4)
  line L4 (0, 4) -> (0, 0)
  line L5 (30.5, -25) -> (18.5, -25)
  line L6 (18.5, -25) -> (18.5, -15)
  line L7 (18.5, -15) -> (30.5, -15)
  line L8 (30.5, -15) -> (30.5, -25)
  line L9 (18.5, -15) -> (12, -15)
  line L10 (12, -15) -> (12, -18)
  line L11 (12, -18) -> (18.5, -18)
  line L12 (18.5, -18) -> (18.5, -15)
  line L13 (18.5, -25) -> (12, -25)
  line L14 (12, -25) -> (12, -22)
  line L15 (12, -22) -> (18.5, -22)
  line L16 (18.5, -22) -> (18.5, -25)
  line L17 (9, 4) -> (9, -2)
  line L18 (12, 4) -> (12, -5)
  dimension "d157" = 3
  dimension "d158" = 3
  constraint horizontal L9
  constraint vertical L10
  constraint horizontal L11
  constraint vertical L12
  constraint coincident L6.end L7.start
  constraint horizontal L13
  constraint vertical L14
  constraint horizontal L15
  constraint vertical L16
  constraint coincident L5.end L6.start
  constraint collinear L10 L14
  constraint collinear L10 L18
  measures "d157" distance of L9.end L10.end
  measures "d158" distance of L13 L15
extrude "Extrude39" add sketch "Sketch40" along normal blind 9 contours L6 L13 L14 L15 L16 | L6 L9 L10 L11 L12 bodies 1
sketch "Sketch41" plane through (70, 0, 0) normal (-1, 0, 0) x (0, -1, 0)
  line L0 (18.5, -22) -> (12, -22)
  line L1 (12, -22) -> (12, -25)
  line L2 (12, -25) -> (18.5, -25)
  line L3 (18.5, -25) -> (18.5, -22)
  line L4 (12, -25) -> (18.5, -25)
  line L5 (18.5, -25) -> (18.5, -15)
  line L6 (18.5, -15) -> (12, -15)
  line L7 (12, -15) -> (12, -25)
  line L8 (18.5, -15) -> (12, -15)
  line L9 (18.5, -18) -> (18.5, -15)
  constraint horizontal L4
  constraint vertical L5
  constraint horizontal L6
  constraint vertical L7
  constraint coincident L1.end L2.start
  constraint collinear L6 L8
  constraint collinear L5 L9
extrude "Extrude40" add sketch "Sketch41" against normal blind 3 bodies 1
equation "d2 = 94 mm - 16 mm"
equation "d5 = 10 mm + 2 mm"
equation "d62 = 29.5 mm + 1 mm"
equation "d66 = 16.5 mm + 4 mm"
equation "d67 = ( 20.5 * 2 ) * 1 mm"
equation "d74 = ( ( 24 + 8.5 + 20 + 4 ) * 2 ) * 1 mm"
equation "d75 = 24 mm + 8.5 mm + 10 mm"
equation "d76 = ( ( 113 / 2 ) * 1 mm )"
equation "d77 = ( ( 113 / 2 ) * 1 mm )"
equation "d95 = 4 mm + 1.5 mm"
equation "d103 = -( 29 mm - 16 mm )"
named bodies: "Sorting Mechanism Platform", "Sorting mechanism platform", "Colour sensor holder"
